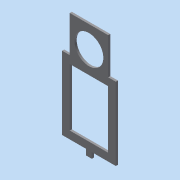
# Autodesk Inventor part: anillo
Saved by Autodesk Inventor 2015 (Build 190159000, 159)
## iProperties
Created: 2017-09-29
Part Number: anillo
Material: Generic
Document SubType Name: Modeling
Designer: macbook
Density: 1 g/cm^3
Appearance: Default
Author: macbook
Autodesk Inventor part; units mm, degrees
ref_plane "YZ Plane" through (0, 0, 0) normal (1, 0, 0) x (0, 1, 0)
ref_plane "XZ Plane" through (0, 0, 0) normal (0, 1, 0) x (-1, 0, 0)
ref_plane "XY Plane" through (0, 0, 0) normal (0, 0, 1) x (1, 0, 0)
sketch "Sketch1" plane through (0, 0, 0) normal (0, 0, 1) x (1, 0, 0)
  line L0 (0, 0) -> (100, 0)
  line L1 (100, 0) -> (100, 150)
  line L2 (100, 150) -> (0, 150)
  line L3 (0, 150) -> (0, 0)
  circle A0 centre (50, 207.5) radius 37.5
  line L4 (-20, -20) -> (120, -20)
  line L5 (120, -20) -> (120, 170)
  line L6 (120, 170) -> (-20, 170)
  line L7 (-20, 170) -> (-20, -20)
  line L8 (0, 170) -> (100, 170)
  line L9 (100, 170) -> (100, 265)
  line L10 (100, 265) -> (0, 265)
  line L11 (0, 265) -> (0, 170)
  line L12 (49.5, -20) -> (59.5, -20)
  line L13 (45, -20) -> (60, -20)
  line L14 (42.5, -20) -> (57.5, -20)
  line L15 (57.5, -20) -> (57.5, -35)
  line L16 (57.5, -35) -> (42.5, -35)
  line L17 (42.5, -35) -> (42.5, -20)
  dimension "d4" = 75
  dimension "d5" = 140
  dimension "d6" = 95
  dimension "d13" = 15
  dimension "d14" = 15
  constraints: 36 end point, 8 parallel, 6 horizontal, 4 perpendicular, 4 point on line, 1 centre point
  measures "d4" diameter of A0
  measures "d5" distance of L6.end L5.end
  measures "d6" distance of L9.end L8.end
  measures "d13" distance of L15.end L16.end
  measures "d14" distance of L14.end L15.end
extrude "Extrusion1" add sketch "Sketch1" along normal blind 5.5
body "Solid1"
